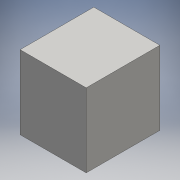
# Autodesk Inventor part: Part2
Saved by Autodesk Inventor 2016 (Build 200138000, 138)
## iProperties
Created: 2018-07-11
Part Number: Part2
Material: Generic
Document SubType Name: Modeling
Designer: olivi
Density: 1 g/cm^3
Appearance: Default
Author: olivi
Autodesk Inventor part; units mm, degrees
ref_plane "YZ Plane" through (0, 0, 0) normal (1, 0, 0) x (0, 1, 0)
ref_plane "XZ Plane" through (0, 0, 0) normal (0, 1, 0) x (-1, 0, 0)
ref_plane "XY Plane" through (0, 0, 0) normal (0, 0, 1) x (1, 0, 0)
sketch "Sketch1" plane through (0, 0, 0) normal (0, 1, 0) x (-1, 0, 0)
  line L0 (110.6195, 133.4808) -> (-113.5693, 133.4808)
  line L1 (-113.5693, 133.4808) -> (-113.5693, -116.5192)
  line L2 (-113.5693, -116.5192) -> (110.6195, -116.5192)
  line L3 (110.6195, -116.5192) -> (110.6195, 133.4808)
  point P0 (0, 0)
  dimension "d0" = 250
  constraints: 8 end point, 2 parallel, 1 horizontal, 1 perpendicular
  measures "d0" distance of L2.end L0.start
extrude "Extrusion1" add sketch "Sketch1" along normal blind 250
body "Solid1"
